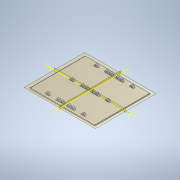
# Autodesk Inventor part: Deckel_PV_Elektronik
Saved by Autodesk Inventor 2021 (Build 250183000, 183)
## iProperties
Created: 2023-10-27
Part Number: Deckel_PV_Elektronik
Material: Generisch
Document SubType Name: Modeling
Designer: pasca
Density: 1 g/cm^3
Appearance: Vorgabe
Author: pasca
Autodesk Inventor part; units mm, degrees
sketch "Skizze1" plane through (0, 0, 0) normal (0, 0, 1) x (1, 0, 0)
  line L0 (-107, -91) -> (107, -91)
  line L1 (107, -91) -> (107, 91)
  line L2 (107, 91) -> (-107, 91)
  line L3 (-107, 91) -> (-107, -91)
  line L4 (0, -127.4) -> (0, 127.4) projected
  line L5 (-149.8, 0) -> (149.8, 0) projected
  point P0 (0, 0)
  dimension "d0" = 182
  dimension "d1" = 214
  constraints: 8 end point, 2 parallel, 1 horizontal, 1 perpendicular, 2 other
  measures "d0" distance between parallel lines of L0 L2
  measures "d1" distance between parallel lines of L1 L3
extrude "Extrusion1" add sketch "Skizze1" against normal blind 3
sketch "Skizze2" plane through (0, 0, 0) normal (0, 1, 0) x (-1, 0, 0)
  line L0 (-107, 0) -> (107, 0) projected
  circle A0 centre (59, 1.9996) radius 1.65
  circle A1 centre (59, 1.9996) radius 4
  line L1 (66, 0) -> (62.0313, 4.6095)
  line L2 (52, 0) -> (55.9688, 4.6095)
  point P0 (0, 0)
  point P1 (-11, 0)
  point P2 (-24, 0)
  point P3 (-59, 0)
  point P4 (59, 0)
  point P5 (24, 0)
  point P6 (11, 0)
  dimension "d4" = 3.3
  dimension "d5" = 8
  constraints: 4 end point, 2 centre point, 2 point on circle, 2 tangent, 1 coincident, 9 other
  measures "d4" diameter of A0
  measures "d5" diameter of A1
extrude "Extrusion2" add sketch "Skizze2" against normal mid plane 6 contours L2 A1 L0 | A1 L0 | A1 L1 L0 picked at (59.0663, 0.1205)
pattern_linear "Rechteckige Anordnung3" count 2 spacing 35 along (1, 0, 0) count 2 spacing 80 along (0, -1, 0) of "Extrusion2"
pattern_linear "Rechteckige Anordnung4" count 2 spacing 35 along (1, 0, 0) count 2 spacing 80 along (0, 1, 0) of "Extrusion2"
pattern_linear "Rechteckige Anordnung5" count 2 spacing 48 along (1, 0, 0) count 2 spacing 80 along (0, -1, 0) of "Extrusion2" second direction both ways yes
pattern_linear "Rechteckige Anordnung6" count 2 spacing 48 along (1, 0, 0) count 2 spacing 80 along (0, 1, 0) of "Extrusion2"
mirror "Spiegeln1" about plane through (0, 0, 0) normal (1, 0, 0) of "Extrusion2", "Rechteckige Anordnung4", "Rechteckige Anordnung6", "Rechteckige Anordnung5", "Rechteckige Anordnung3"
sketch "Skizze3" plane through (0, 0, 0) normal (0, 1, 0) x (-1, 0, 0)
  line L0 (-107, 0) -> (107, 0) projected
  circle A0 centre (106.5, 0) radius 0.5
  line L1 (0, -4.7999) -> (0, 7.7995) projected
  point P0 (0, 0)
  point P1 (106, 0)
  dimension "d38" = 1
  dimension "d39" = 106.5
  constraints: 1 centre point, 1 point on line
  measures "d38" diameter of A0
  measures "d39" distance from line of L1 A0.centre
extrude "Extrusion3" add sketch "Skizze3" along normal mid plane 180 contours A0 L0 picked at (106.6248, 0.1903)
mirror "Spiegeln2" about plane through (0, 0, 0) normal (1, 0, 0) of "Extrusion3"
sketch "Skizze4" plane through (0, 0, 0) normal (0, 0, 1) x (1, 0, 0)
  line L0 (-149.8, 0) -> (149.8, 0) projected
  line L1 (0, 127.4) -> (0, -127.4) projected
  point P0 (0, 0)
ref_plane "Arbeitsebene1" through (0, 0, 0) normal (1, 0, 0) x (0, 1, 0)
